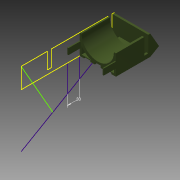
# Autodesk Inventor part: 知能ロボコン発射台２.1
Saved by Autodesk Inventor 2013 (Build 170138000, 138)
## iProperties
Created: 2014-05-17
Part Number: 知能ロボコン発射台２.1
Material: ABS プラスチック
Document SubType Name: Modeling
Designer: horumo136
Density: 1.06 g/cm^3
Mass: 430.971 g
Surface Area: 1189.26 cm^2
Volume: 406.576 cm^3
Author: horumo136
Autodesk Inventor part; units mm, degrees
ref_plane "YZ Plane" through (0, 0, 0) normal (1, 0, 0) x (0, 1, 0)
ref_plane "XZ Plane" through (0, 0, 0) normal (0, 1, 0) x (-1, 0, 0)
ref_plane "XY Plane" through (0, 0, 0) normal (0, 0, 1) x (1, 0, 0)
sketch "スケッチ1" plane through (0, 0, 0) normal (0, 1, 0) x (-1, 0, 0)
  line L0 (0, 0) -> (-90, 0)
  line L1 (-90, 0) -> (-90, 50)
  line L2 (0, 50) -> (0, 0)
  line L3 (0, 0) -> (-5, 0)
  line L4 (-5, 0) -> (-5, 50)
  line L5 (-5, 0) -> (-90, 0)
  line L6 (-90, 0) -> (-85, 0)
  line L7 (-85, 0) -> (-85, 50)
  arc A0 (-85, 50) -> (-5, 50) centre (-45, 50) ccw
  line L8 (0, 0) -> (0, 10)
  line L9 (0, 10) -> (-90, 10)
  circle A1 centre (-45, 50) radius 45
  line L10 (-90, 5) -> (0, 5)
  line L11 (-90, 50) -> (-85, 50)
  line L12 (-5, 50) -> (0, 50)
  line L13 (0, 0) -> (-90, 0)
  line L14 (-90, 0) -> (-90, 5)
  line L15 (-90, 5) -> (0, 5)
  line L16 (0, 5) -> (0, 0)
  dimension "d0" = 90
  dimension "d1" = 50
  dimension "d2" = 5
  dimension "d3" = 85
  dimension "d4" = 5
  dimension "d5" = 80
  dimension "d6" = 10
  dimension "d7" = 90
  constraints: 34 end point, 7 perpendicular, 5 parallel, 5 point on line, 2 centre point, 2 horizontal, 2 point on circle, 1 coincident, 1 collinear, 1 midpoint
  measures "d0" distance of L1.end L2.start
  measures "d1" distance of L0.end L1.end
  measures "d2" distance of L0.start L3.end
  measures "d3" distance of L3.end L0.end
  measures "d4" distance of L0.end L6.end
  measures "d5" diameter of A0
  measures "d6" distance of L0.start L8.end
  measures "d7" diameter of A1
extrude "押し出し1" add sketch "スケッチ1" along normal blind 230 contours L0 L4 L10 L2 | L0 L7 L10 L4 | L10 L4 L9 L2 | L0 L1 L10 L7 | L10 A1 L9 L4 | L9 L4 A1 L2 | L10 L1 L9 L7 | L7 L9 A1 L10 | L9 A1 L4 | A1 L9 | A1 L4 L12 | L9 L1 A1 L7 | L7 A1 L9 | A1 L9 A0 L4 | A1 L7 A0 L9 | L11 L7 A1
sketch "スケッチ2" plane through (0, 0, 0) normal (0, -1, 0) x (1, 0, 0)
  line L0 (0, 0) -> (0, 50) projected
  line L1 (90, 0) -> (0, 0) projected
  line L2 (90, 50) -> (90, 0) projected
  line L3 (85, 50) -> (90, 50) projected
  arc A0 (5, 50) -> (85, 50) centre (45, 50) ccw projected
  line L4 (0, 50) -> (5, 50) projected
  arc A1 (5, 23.467) -> (85, 23.467) centre (45, 50) ccw
  line L5 (0, 5) -> (90, 5)
  line L6 (5, 23.467) -> (5, 5)
  line L7 (85, 23.467) -> (85, 5)
  dimension "d29" = 48
  constraints: 8 end point, 4 point on line, 3 perpendicular, 2 point on circle, 2 tangent, 1 centre point, 1 coincident
  measures "d29" radius of A1
extrude "押し出し2" cut sketch "スケッチ2" against normal blind 225 contours L6 A1 L5 | L5 A1 L7
sketch "スケッチ3" plane through (0, 230, 0) normal (0, 1, 0) x (1, 0, 0)
  arc A0 (85, -50) -> (5, -50) centre (45, -50) ccw projected
  line L0 (90, -50) -> (90, 0) projected
  line L1 (0, -50) -> (5, -50) projected
  arc A1 (85, -50) -> (5, -50) centre (45, -50) ccw
  line L2 (5, -50) -> (85, -50)
  constraints: 3 end point, 2 point on circle, 1 centre point, 1 coincident, 1 perpendicular
extrude "押し出し3" add sketch "スケッチ3" against normal blind 5
sketch "スケッチ4" plane through (90, 0, 50) normal (1, 0, 0) x (0, 0, -1)
  line L0 (0, 0) -> (50, 0) projected
  line L1 (0, 0) -> (0, 230) projected
  line L2 (25, 0) -> (25, 65)
  line L3 (25, 65) -> (25, 75)
  line L4 (25, 75) -> (25, 215)
  line L5 (25, 215) -> (25, 225)
  line L6 (0, 65) -> (40, 65)
  line L7 (40, 65) -> (40, 75)
  line L8 (40, 75) -> (0, 75)
  line L9 (0, 75) -> (0, 65)
  line L10 (0, 215) -> (40, 215)
  line L11 (40, 215) -> (40, 225)
  line L12 (40, 225) -> (0, 225)
  line L13 (0, 225) -> (0, 215)
  dimension "d16" = 65
  dimension "d17" = 10
  dimension "d18" = 140
  dimension "d19" = 10
  dimension "d20" = 40
  constraints: 24 end point, 5 parallel, 3 collinear, 2 horizontal, 2 perpendicular, 2 point on line, 1 midpoint
  measures "d16" distance of L2.start L2.end
  measures "d17" distance of L2.end L3.end
  measures "d18" distance of L3.end L4.end
  measures "d19" distance of L4.end L5.end
  measures "d20" distance of L8.end L7.end
extrude "押し出し4" cut sketch "スケッチ4" against normal blind 90 contours L1 L8 L3 L6 | L3 L8 L7 L6 | L1 L12 L5 L10 | L5 L12 L11 L10
sketch "スケッチ6" plane through (90, 0, 50) normal (1, 0, 0) x (0, 0, -1)
  line L0 (0, 230) -> (50, 230) projected
  line L1 (50, 230) -> (37.5, 251.6506)
  line L2 (50, 230) -> (110, 230) construction
  line L3 (0, 230) -> (37.5, 251.6506)
  line L4 (0, 230) -> (43.3013, 230) construction
  dimension "d32" = 120
  dimension "d33" = 30
  constraints: 8 end point, 2 horizontal, 1 equal length
  measures "d32" angle of L2 L1
  measures "d33" angle of L4 L3
extrude "押し出し6" add sketch "スケッチ6" against normal blind 90
sketch "スケッチ9" plane through (0, 0, 0) normal (-1, 0, 0) x (0, 0, 1)
  line L0 (10, 225) -> (50, 225) projected
  line L1 (50, 225) -> (50, 230) projected
  line L2 (50, 230) -> (12.5, 251.6506) projected
  line L3 (12.5, 251.6506) -> (0, 230) projected
  line L4 (0, 0) -> (0, 230) projected
  line L5 (0, 0) -> (50, 0) projected
  line L6 (50, 0) -> (50, 65) projected
  line L7 (50, 65) -> (10, 65) projected
  line L8 (10, 65) -> (10, 75) projected
  line L9 (10, 75) -> (50, 75) projected
  line L10 (50, 75) -> (50, 215) projected
  line L11 (50, 215) -> (10, 215) projected
  line L12 (10, 215) -> (10, 225) projected
  line L13 (12.5, 251.6506) -> (0, 230)
  line L14 (0, 230) -> (-132.7906, 0)
  line L15 (0, 145) -> (-49.0748, 145)
  line L16 (0, 115) -> (-66.3953, 115)
  dimension "d45" = 30
  constraints: 8 end point, 2 collinear, 2 midpoint, 2 point on line, 1 perpendicular
  measures "d45" distance between parallel lines of L15 L16
sketch "スケッチ10" plane through (0, 0, 0) normal (-1, 0, 0) x (0, 0, 1)
  line L0 (10, 225) -> (50, 225) projected
  line L1 (50, 225) -> (50, 230) projected
  line L2 (50, 230) -> (12.5, 251.6506) projected
  line L3 (12.5, 251.6506) -> (0, 230) projected
  line L4 (0, 0) -> (0, 230) projected
  line L5 (0, 0) -> (50, 0) projected
  line L6 (50, 0) -> (50, 65) projected
  line L7 (50, 65) -> (10, 65) projected
  line L8 (10, 65) -> (10, 75) projected
  line L9 (10, 75) -> (50, 75) projected
  line L10 (50, 75) -> (50, 215) projected
  line L11 (50, 215) -> (10, 215) projected
  line L12 (10, 215) -> (10, 225) projected
  line L13 (12.5, 251.6506) -> (-87.5, 78.4456)
  line L14 (-87.5, 78.4456) -> (50, 0)
  constraints: 4 end point, 1 collinear
sketch "スケッチ11" plane through (90, 230, 0) normal (0, 0.5, -0.866) x (-1, 0, 0)
  line L0 (0, 25) -> (90, 25) projected
  line L1 (45, 25) -> (45, 15)
  line L2 (45, 15) -> (60, 15)
  line L3 (60, 15) -> (30, 15)
  point P0 (90, -199.1858)
  dimension "d49" = 10
  dimension "d50" = 15
  dimension "d51" = 30
  constraints: 6 end point, 4 coincident, 2 perpendicular, 1 collinear, 1 midpoint
  measures "d49" distance of L1.start L1.end
  measures "d50" distance of L1.end L2.end
  measures "d51" distance of L2.end L3.end
hole "穴1" at (45, 242.9904, 7.5) at (30, 242.9904, 7.5) at (60, 242.9904, 7.5) direction (0, -0.5, 0.866) diameter 2.5 depth 8 tip angle 118
sketch "スケッチ12" plane through (90, 0, 50) normal (1, 0, 0) x (0, 0, -1)
  line L0 (50, 0) -> (50, 230) projected
  line L1 (40, 225) -> (40, 215) projected
  line L2 (0, 215) -> (0, 75)
  line L3 (0, 145) -> (50, 145)
  line L4 (32.5, 175) -> (17.5, 175)
  line L5 (17.5, 175) -> (17.5, 115)
  line L6 (17.5, 115) -> (32.5, 115)
  line L7 (32.5, 115) -> (32.5, 175)
  line L8 (32.5, 175) -> (17.5, 115) construction
  line L9 (17.5, 175) -> (32.5, 115) construction
  line L10 (17.5, 145) -> (32.5, 145)
  line L11 (32.5, 145) -> (32.5, 115)
  line L12 (32.5, 115) -> (17.5, 115)
  line L13 (17.5, 115) -> (17.5, 145)
  point P0 (25, 145)
  dimension "d59" = 15
  dimension "d60" = 60
  constraints: 24 end point, 5 midpoint, 5 parallel, 3 perpendicular, 2 horizontal, 1 point on line
  measures "d59" distance of L6.end L5.end
  measures "d60" distance of L5.end L4.end
extrude "押し出し8" cut sketch "スケッチ12" against normal blind 2.5 contours L3 L7 L6 L5
sketch "スケッチ13" plane through (0, 0, 0) normal (-1, 0, 0) x (0, 0, 1)
  line L0 (0, 0) -> (0, 230) projected
  line L1 (50, 75) -> (50, 215) projected
  line L2 (50, 145) -> (0, 145)
  line L3 (17.5, 175) -> (32.5, 175)
  line L4 (32.5, 175) -> (32.5, 115)
  line L5 (32.5, 115) -> (17.5, 115)
  line L6 (17.5, 115) -> (17.5, 175)
  line L7 (17.5, 175) -> (32.5, 115) construction
  line L8 (32.5, 175) -> (17.5, 115) construction
  line L9 (17.5, 145) -> (32.5, 145)
  line L10 (32.5, 145) -> (32.5, 115)
  line L11 (32.5, 115) -> (17.5, 115)
  line L12 (17.5, 115) -> (17.5, 145)
  point P0 (25, 145)
  dimension "d63" = 15
  dimension "d64" = 60
  constraints: 22 end point, 5 midpoint, 4 parallel, 3 perpendicular, 2 horizontal, 1 point on line
  measures "d63" distance of L4.end L5.end
  measures "d64" distance of L3.end L4.end
extrude "押し出し9" cut sketch "スケッチ13" against normal blind 2.5 contours L4 L5 L6 L2
sketch "スケッチ14" plane through (90, 0, 0) normal (0, 0, -1) x (-1, 0, 0)
  line L0 (90, 0) -> (90, 230) projected
  line L1 (0, 0) -> (0, 230) projected
  line L2 (0, 145) -> (90, 145)
  line L3 (37.5, 170) -> (52.5, 170)
  line L4 (52.5, 170) -> (52.5, 120)
  line L5 (52.5, 120) -> (37.5, 120)
  line L6 (37.5, 120) -> (37.5, 170)
  line L7 (37.5, 170) -> (52.5, 120) construction
  line L8 (52.5, 170) -> (37.5, 120) construction
  line L9 (37.5, 145) -> (52.5, 145)
  line L10 (52.5, 145) -> (52.5, 170)
  line L11 (52.5, 170) -> (37.5, 170)
  line L12 (37.5, 170) -> (37.5, 145)
  point P0 (45, 145)
  dimension "d67" = 15
  dimension "d70" = 25
  constraints: 22 end point, 4 midpoint, 4 parallel, 3 perpendicular, 2 horizontal, 2 point on line
  measures "d67" distance of L4.end L5.end
  measures "d70" distance of L11.end L9.start
extrude "押し出し10" cut sketch "スケッチ14" against normal blind 5 contours L6 L3 L4 L2
sketch "スケッチ16" plane through (90, 0, 0) normal (0, 0, -1) x (-1, 0, 0)
  line L0 (52.5, 170) -> (52.5, 145) projected
  line L1 (52.5, 145) -> (37.5, 145) projected
  line L2 (37.5, 145) -> (37.5, 170) projected
  line L3 (90, 0) -> (90, 230) projected
  line L4 (0, 0) -> (0, 230) projected
  line L5 (0, 145) -> (90, 145)
  line L6 (0, 160) -> (37.5, 157.5)
  line L7 (52.5, 157.5) -> (90, 157.5)
  line L8 (18.75, 158.75) -> (18.75, 145)
  line L9 (71.25, 145) -> (71.25, 157.5)
  line L10 (11.25, 175) -> (26.25, 175)
  line L11 (26.25, 175) -> (26.25, 115)
  line L12 (26.25, 115) -> (11.25, 115)
  line L13 (11.25, 115) -> (11.25, 175)
  line L14 (11.25, 175) -> (26.25, 115) construction
  line L15 (26.25, 175) -> (11.25, 115) construction
  line L16 (11.25, 115) -> (26.25, 115)
  line L17 (26.25, 115) -> (26.25, 175)
  line L18 (26.25, 175) -> (11.25, 175)
  line L19 (11.25, 175) -> (11.25, 115)
  line L20 (45, 145) -> (45, 125)
  line L21 (78.75, 175) -> (63.75, 175)
  line L22 (63.75, 115) -> (78.75, 115)
  line L23 (78.75, 175) -> (78.75, 115)
  line L24 (63.75, 115) -> (63.75, 175)
  line L25 (63.75, 175) -> (78.75, 175)
  line L26 (78.75, 175) -> (78.75, 115)
  line L27 (78.75, 115) -> (63.75, 115)
  line L28 (63.75, 115) -> (63.75, 175)
  line L29 (11.25, 115) -> (26.25, 115)
  line L30 (26.25, 115) -> (26.25, 175)
  line L31 (26.25, 175) -> (11.25, 175)
  line L32 (11.25, 175) -> (11.25, 115)
  dimension "d71" = 15
  dimension "d72" = 60
  dimension "d73" = 20
  constraints: 56 end point, 12 symmetric about line, 7 midpoint, 7 perpendicular, 6 parallel, 6 point on line, 3 horizontal
  measures "d71" distance of L11.end L12.end
  measures "d72" distance of L10.end L11.end
  measures "d73" distance of L20.start L20.end
extrude "押し出し11" cut sketch "スケッチ16" against normal blind 3 contours L24 L21 L23 L7 | L7 L9 L5 L24 | L5 L23 L22 L24 | L7 L23 L5 L9 | L11 L12 L13 L5 | L5 L8 L6 L11 | L6 L13 L10 L11 | L5 L13 L6 L8
sketch "スケッチ17" plane through (37.5, 145, 0) normal (0, 1, 0) x (1, 0, 0)
  line L0 (-57.7643, 16.522) -> (69.053, 16.522)
  line L1 (69.053, 16.522) -> (69.053, -65.9751)
  line L2 (69.053, -65.9751) -> (-57.7643, -65.9751)
  line L3 (-57.7643, -65.9751) -> (-57.7643, 16.522)
  point P0 (-37.5, 0)
  constraints: 8 end point, 2 parallel, 1 horizontal, 1 perpendicular
extrude "押し出し12" cut sketch "スケッチ17" against normal blind 180
sketch "スケッチ18" plane through (0, 215, 10) normal (-1, 0, 0) x (0, 0, 1)
  line L0 (-10, -70) -> (40, -70) projected
  line L1 (7.5, -40) -> (22.5, -40)
  line L2 (22.5, -40) -> (22.5, -100)
  line L3 (22.5, -100) -> (7.5, -100)
  line L4 (7.5, -100) -> (7.5, -40)
  line L5 (7.5, -40) -> (22.5, -100) construction
  line L6 (22.5, -40) -> (7.5, -100) construction
  point P0 (-10, -215)
  point P1 (15, -70)
  dimension "d78" = 15
  dimension "d79" = 60
  constraints: 12 end point, 3 midpoint, 2 parallel, 1 horizontal, 1 perpendicular
  measures "d78" distance of L2.end L3.end
  measures "d79" distance of L1.end L2.end
extrude "押し出し13" add sketch "スケッチ18" against normal blind 2.5
sketch "スケッチ19" plane through (90, 215, 10) normal (1, 0, 0) x (0, 0, -1)
  line L0 (-40, -70) -> (10, -70) projected
  line L1 (-22.5, -40) -> (-7.5, -40)
  line L2 (-7.5, -40) -> (-7.5, -100)
  line L3 (-7.5, -100) -> (-22.5, -100)
  line L4 (-22.5, -100) -> (-22.5, -40)
  line L5 (-22.5, -40) -> (-7.5, -100) construction
  line L6 (-7.5, -40) -> (-22.5, -100) construction
  point P0 (10, -215)
  point P1 (-15, -70)
  dimension "d82" = 15
  dimension "d83" = 60
  constraints: 12 end point, 3 midpoint, 2 parallel, 1 horizontal, 1 perpendicular
  measures "d82" distance of L2.end L3.end
  measures "d83" distance of L1.end L2.end
extrude "押し出し14" add sketch "スケッチ19" against normal blind 2.5
